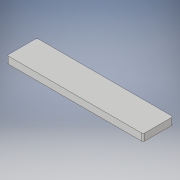
# Autodesk Inventor part: Stapler
Saved by Autodesk Inventor 2017 (Build 210142000, 142)
## iProperties
Created: 2018-03-21
Part Number: Stapler
Material: Generic
Document SubType Name: Modeling
Designer: landontracy
Density: 1 g/cm^3
Appearance: Default
Author: landontracy
Autodesk Inventor part; units mm, degrees
ref_plane "YZ Plane" through (0, 0, 0) normal (1, 0, 0) x (0, 1, 0)
ref_plane "XZ Plane" through (0, 0, 0) normal (0, 1, 0) x (-1, 0, 0)
ref_plane "XY Plane" through (0, 0, 0) normal (0, 0, 1) x (1, 0, 0)
sketch "Stapler Bottom" plane through (0, 0, 0) normal (0, 1, 0) x (-1, 0, 0)
  line L0 (94.8504, -32.7544) -> (-89.2889, -32.7544)
  line L1 (-90.2889, -31.6958) -> (-90.2889, 7.1831)
  line L2 (-89.8327, 8.1831) -> (94.7084, 8.1831)
  line L3 (95.8504, 7.1831) -> (95.8504, -30.3771)
  line L4 (95.8504, 7.1831) -> (94.7084, 8.1831)
  line L5 (95.8504, -30.3771) -> (94.8504, -32.7544)
  line L6 (-89.2889, -32.7544) -> (-90.2889, -31.6958)
  line L7 (-90.2889, 7.1831) -> (-89.8327, 8.1831)
  point P0 (0, 0)
  dimension "d2" = 1
  dimension "d3" = 1
  dimension "d4" = 1
  dimension "d5" = 1
  dimension "d6" = 38.8788
  dimension "d7" = 184.5411
  constraints: 16 end point, 2 parallel, 1 horizontal, 1 perpendicular
  measures "d2" vertical distance of L3.start L2.end
  measures "d3" horizontal distance of L3.end L0.start
  measures "d4" horizontal distance of L0.end L1.start
  measures "d5" vertical distance of L1.end L2.start
  measures "d6" distance of L1.start L1.end
  measures "d7" distance of L2.start L2.end
extrude "Extrusion1" add sketch "Stapler Bottom" along normal blind 9.52
fillet "Fillet1" radius 2 8 edges at (89.8327, 4.76, 8.1831) (90.2889, 4.76, 7.1831) (89.2889, 4.76, -32.7544) (90.2889, 4.76, -31.6958) (-94.8504, 4.76, -32.7544) (-95.8504, 4.76, -30.3771) (-95.8504, 4.76, 7.1831) (-94.7084, 4.76, 8.1831)
body "Solid1"
